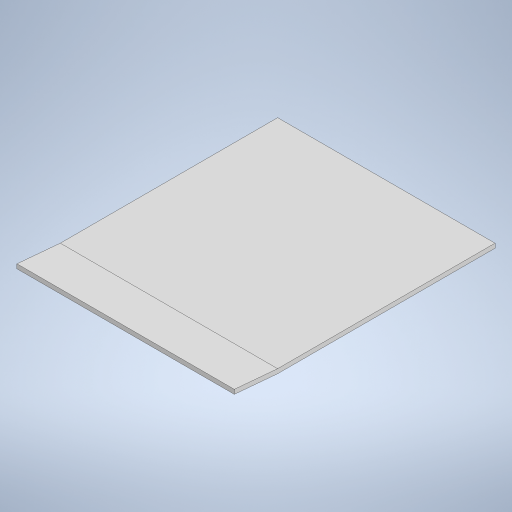
# Autodesk Inventor part: NHK_t0_15
Saved by Autodesk Inventor 2023 (Build 270158000, 158)
## iProperties
Created: 2022-04-18
Part Number: NHK_t0_15
Material: 一般
Document SubType Name: Modeling
Designer: yuta
Density: 1 g/cm^3
Appearance: 既定
Author: yuta
Autodesk Inventor part; units mm, degrees
ref_plane "YZ Plane" through (0, 0, 0) normal (1, 0, 0) x (0, 1, 0)
ref_plane "XZ Plane" through (0, 0, 0) normal (0, 1, 0) x (-1, 0, 0)
ref_plane "XY Plane" through (0, 0, 0) normal (0, 0, 1) x (1, 0, 0)
sketch "スケッチ1" plane through (0, 0, 0) normal (1, 0, 0) x (0, 1, 0)
  line L0 (0, 0) -> (2.6147, 29.8858)
  line L1 (0, 0) -> (30, 0) construction
  line L2 (2.6147, 29.8858) -> (5.6147, 29.8858)
  line L3 (5.6147, 29.8858) -> (3, 0)
  line L4 (3, 0) -> (0, 0)
  dimension "d0" = 30
  dimension "d1" = 85
  dimension "d2" = 3
  dimension "d3" = 95
  dimension "d4" = 30
  dimension "d5" = 85
  constraints: 10 end point, 2 horizontal, 1 equal length, 1 parallel
  measures "d0" distance of L0.start L0.end
  measures "d1" angle of L1 L0
  measures "d2" distance of L0.end L2.end
  measures "d3" angle of L0 L2
  measures "d4" distance of L2.end L3.end
  measures "d5" angle of L2 L3
sketch "スケッチ2" plane through (0, 0, 0) normal (1, 0, 0) x (0, 1, 0)
  point P0 (0, 0)
extrude "押し出し1" add sketch "スケッチ1" along normal blind 150
sketch "スケッチ3" plane through (150, 0, 0) normal (1, 0, 0) x (0, 0, -1)
  line L0 (0, 0) -> (150, 0)
  line L1 (150, 0) -> (150, 3)
  line L2 (150, 3) -> (0, 3)
  line L3 (0, 3) -> (0, 0)
  dimension "d8" = 150
  dimension "d9" = 3
  constraints: 8 end point, 2 parallel, 1 horizontal, 1 perpendicular
  measures "d8" distance of L2.end L1.end
  measures "d9" distance of L1.end L0.end
extrude "押し出し2" add sketch "スケッチ3" against normal blind 150
